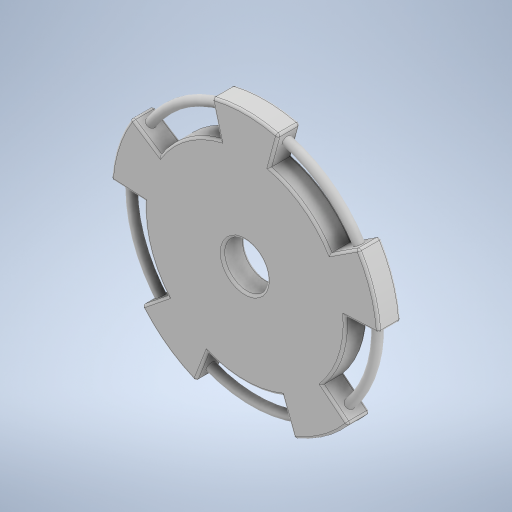
# Autodesk Inventor part: structure
Saved by Autodesk Inventor 2024 (Build 280153000, 153)
## iProperties
Created: 2023-05-06
Part Number: structure
Material: Generic
Document SubType Name: Modeling
Designer: Sujith
Density: 1 g/cm^3
Appearance: Default
Author: Sujith
Autodesk Inventor part; units mm, degrees
ref_plane "YZ Plane" through (0, 0, 0) normal (1, 0, 0) x (0, 1, 0)
ref_plane "XZ Plane" through (0, 0, 0) normal (0, 1, 0) x (-1, 0, 0)
ref_plane "XY Plane" through (0, 0, 0) normal (0, 0, 1) x (1, 0, 0)
sketch "Sketch1" plane through (0, 0, 0) normal (0, 0, 1) x (1, 0, 0)
  circle A0 centre (0, 0) radius 5
  circle A1 centre (0, 0) radius 30
  circle A2 centre (0, 0) radius 22.5
  line L0 (-5.5294, 21.81) -> (-7.4706, 29.0549)
  line L1 (5.5294, 21.81) -> (7.4706, 29.0549)
  line L2 (0, 30) -> (0, -30) construction
  line L3 (-43.3473, 0) -> (46.0225, 0) construction
  line L4 (-22.4512, 1.4809) -> (-29.9414, 1.8735)
  line L5 (-19.0339, 11.9984) -> (-25.3243, 16.0835)
  line L6 (-8.3462, -20.8947) -> (-11.0342, -27.8971)
  line L7 (-17.2929, -14.3946) -> (-23.1219, -19.1148)
  line L8 (17.2929, -14.3946) -> (23.1219, -19.1148)
  line L9 (8.3462, -20.8947) -> (11.0342, -27.8971)
  line L10 (19.0339, 11.9984) -> (25.3243, 16.0835)
  line L11 (22.4512, 1.4809) -> (29.9414, 1.8735)
  point P0 (6.5, 25.4325)
  point P1 (-6.5, 25.4325)
  point P2 (-26.1963, 1.6772)
  point P3 (-22.1791, 14.0409)
  point P4 (-9.6902, -24.3959)
  point P5 (-20.2074, -16.7547)
  point P6 (20.2074, -16.7547)
  point P7 (9.6902, -24.3959)
  point P8 (22.1791, 14.0409)
  point P9 (26.1963, 1.6772)
  dimension "d0" = 10
  dimension "d1" = 60
  dimension "d3" = 7.5
  dimension "d7" = 30
  dimension "d8" = 13
  dimension "d11" = 360
  constraints: 24 end point, 6 point on circle, 3 centre point, 2 coincident, 2 midpoint, 1 horizontal, 42 other
  measures "d0" diameter of A0
  measures "d1" diameter of A1
  measures "d3" radial gap between concentric circles of A1 A2
  measures "d7" angle of L1 L0
  measures "d8" distance of point (6.5, 25.432) point (-6.5, 25.432)
extrude "Extrusion1" add sketch "Sketch1" along normal mid plane 5 contours L11 A2 L10 A1 | A1 L9 A2 L8 | A2 | L1 A2 L0 A1 | A1 L7 A2 L6 | L5 A2 L4 A1
sketch "Sketch4" plane through (7.4706, 29.0549, 2.5) normal (0.9659258, -0.258819, 0) x (0, 0, -1)
  circle A0 centre (2.5, -2.5) radius 1
  line L0 (5, 0) -> (0, 0) projected
  line L1 (6, -29.9985) -> (-1, -29.9985) projected
  point P0 (2.5, -29.9985)
  point P1 (2.5, 0)
  dimension "d18" = 2
  dimension "d19" = 2.5
  constraints: 1 centre point, 1 midpoint
  measures "d18" diameter of A0
  measures "d19" distance of A0.centre point (2.5, 0)
revolve "Revolution1" add sketch "Sketch4" angle 360 about axis through (-0.2935, 0.0787, -10) along (0, 0, 1)
fillet "Fillet1" radius 0.5 52 edges at (6.5, 25.4325, 2.5) (7.4706, 29.0549, 0) (6.5, 25.4325, -2.5) (22.1791, 14.0409, 2.5) (25.3243, 16.0835, 0) (22.1791, 14.0409, -2.5) (21.3988, -6.9529, 2.5) (20.2074, -16.7547, 2.5) (26.1963, 1.6772, 2.5) (17.6336, -24.2705, 2.5) (28.5317, 9.2705, 2.5) (9.6902, -24.3959, 2.5) (0, -22.5, 2.5) (13.2252, 18.2029, 2.5) (-9.6902, -24.3959, 2.5) (-17.6336, -24.2705, 2.5) (0, 30, 2.5) (-20.2074, -16.7547, 2.5) (-6.5, 25.4325, 2.5) (-21.3988, -6.9529, 2.5) (-13.2252, 18.2029, 2.5) (-26.1963, 1.6772, 2.5) (-22.1791, 14.0409, 2.5) (-28.5317, 9.2705, 2.5) (-5, 0, 2.5) (13.2252, 18.2029, -2.5) (-7.4706, 29.0549, 0) (0, 30, -2.5) (21.3988, -6.9529, -2.5) (20.2074, -16.7547, -2.5) (26.1963, 1.6772, -2.5) (17.6336, -24.2705, -2.5) (28.5317, 9.2705, -2.5) (9.6902, -24.3959, -2.5) (0, -22.5, -2.5) (-9.6902, -24.3959, -2.5) (-17.6336, -24.2705, -2.5) (-20.2074, -16.7547, -2.5) (-6.5, 25.4325, -2.5) (-21.3988, -6.9529, -2.5) (-13.2252, 18.2029, -2.5) (-26.1963, 1.6772, -2.5) (-22.1791, 14.0409, -2.5) (-28.5317, 9.2705, -2.5) (-5, 0, -2.5) (29.9414, 1.8735, 0) (23.1219, -19.1148, 0) (11.0342, -27.8971, 0) (-11.0342, -27.8971, 0) (-23.1219, -19.1148, 0) (-29.9414, 1.8735, 0) (-25.3243, 16.0835, 0)
body "Solid1"
